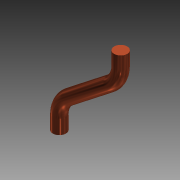
# Autodesk Inventor part: FeedSplitter
Saved by Autodesk Inventor 2014 (Build 180170000, 170)
## iProperties
Created: 2015-05-01
Part Number: FeedSplitter
Material: Generic
Document SubType Name: Modeling
Designer: Owner
Density: 1 g/cm^3
Appearance: Copper - Polished
Author: Owner
Autodesk Inventor part; units mm, degrees
ref_plane "YZ Plane" through (0, 0, 0) normal (1, 0, 0) x (0, 1, 0)
ref_plane "XZ Plane" through (0, 0, 0) normal (0, 1, 0) x (-1, 0, 0)
ref_plane "XY Plane" through (0, 0, 0) normal (0, 0, 1) x (1, 0, 0)
sketch "Sketch1" plane through (0, 0, 0) normal (0, 0, 1) x (1, 0, 0)
  line L0 (0.0306, -0.0109) -> (0.0306, 6.3391)
  line L1 (4.9085, 16.3443) -> (24.9188, 31.9886)
  line L2 (29.7967, 41.9938) -> (29.7967, 48.3438)
  arc A0 (4.9085, 16.3443) -> (0.0306, 6.3391) centre (12.7306, 6.3391) ccw
  arc A1 (24.9188, 31.9886) -> (29.7967, 41.9938) centre (17.0967, 41.9938) ccw
  point P0 (0, 0)
  point P1 (0.0306, 12.5307)
  dimension "d3" = 12.7
  dimension "d4" = 6.35
  dimension "d5" = 6.35
  dimension "d6" = 25.4
  constraints: 6 end point, 4 point on circle, 4 tangent, 2 centre point, 2 point on line, 1 equal radius, 1 parallel, 1 vertical
  measures "d3" radius of A0
  measures "d4" distance of L0.start L0.end
  measures "d5" distance of L2.start L2.end
  measures "d6" distance of L1.start L1.end
sketch "Sketch2" plane through (0, 0, 0) normal (0, 1, 0) x (-1, 0, 0)
  circle A0 centre (0, 0) radius 3.175
  dimension "d1" = 6.35
  constraints: 1 centre point
  measures "d1" diameter of A0
sweep "Sweep1" add profiles "Sketch2" path "Sketch1" path curves L0 A0 L1 A1 L2
body "Solid1"
